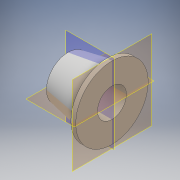
# Autodesk Inventor part: часть шкива
Saved by Autodesk Inventor 2018.3 (Build 223284000, 284)
## iProperties
Created: 2018-12-14
Part Number: часть шкива
Material: Типовые
Document SubType Name: Modeling
Designer: kriku
Density: 1 g/cm^3
Appearance: По умолчанию
Mass: 623.187 g
Surface Area: 736.889 cm^2
Volume: 623.187 cm^3
Author: kriku
Autodesk Inventor part; units mm, degrees
sketch "Эскиз1" plane through (0, 0, 0) normal (0, 0, 1) x (1, 0, 0)
  line L0 (-109.2, 0) -> (18.2, 0) projected
  line L1 (0, 30) -> (-91, 30)
  line L2 (-91, 30) -> (-91, 44.8125)
  line L3 (-91, 44.8125) -> (-10, 60)
  line L4 (-10, 60) -> (-10, 75)
  line L5 (-10, 75) -> (0, 75)
  line L6 (0, 75) -> (0, 30)
  line L7 (0, 90) -> (0, -15) projected
  point P0 (0, 0)
  dimension "d0" = 91
  dimension "d1" = 30
  dimension "d3" = 60
  dimension "d4" = 81
  dimension "d5" = 15
  dimension "d7" = 100.62
  constraints: 12 end point, 3 perpendicular, 1 horizontal, 1 point on line, 1 vertical
  measures "d0" distance of L1.start L1.end
  measures "d1" distance between parallel lines of L0 L1
  measures "d3" distance from line of L0 L3.end
  measures "d4" distance between parallel lines of L2 L4
  measures "d5" distance of L3.end L4.end
  measures "d7" angle of L2 L3
revolve "Вращение1" add sketch "Эскиз1" angle 360 about axis through (0, 0, 0) along (1, 0, 0)
